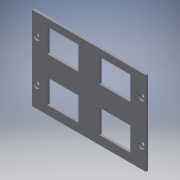
# Autodesk Inventor part: Ra-Manager_Painel-Placas_Tras_Plugs
Saved by Autodesk Inventor 2019.4 (Build 234330000, 330)
## iProperties
Created: 2020-03-24
Part Number: Ra-Manager_Painel-Placas_Tras_Plugs
Material: Genérico
Document SubType Name: Modeling
Designer: caiom
Density: 1 g/cm^3
Appearance: Padrão
Author: caiom
Autodesk Inventor part; units mm, degrees
ref_plane "YZ Plane" through (0, 0, 0) normal (1, 0, 0) x (0, 1, 0)
ref_plane "XZ Plane" through (0, 0, 0) normal (0, 1, 0) x (-1, 0, 0)
ref_plane "XY Plane" through (0, 0, 0) normal (0, 0, 1) x (1, 0, 0)
sketch "Esboço1" plane through (0, 0, 0) normal (0, 0, 1) x (1, 0, 0)
  line L0 (-50.5, -37) -> (50.5, -37)
  line L1 (50.5, -37) -> (50.5, 37)
  line L2 (50.5, 37) -> (-50.5, 37)
  line L3 (-50.5, 37) -> (-50.5, -37)
  point P0 (0, 0)
  point P1 (0, 0)
  dimension "d17" = 101
  dimension "d18" = 74
  dimension "d19" = 50.5
  dimension "d20" = 37
  dimension "d21" = 50.5
  dimension "d22" = 37
  constraints: 8 end point, 2 parallel, 1 perpendicular, 1 vertical
  measures "d17" distance between parallel lines of L1 L3
  measures "d18" distance between parallel lines of L0 L2
  measures "d19" distance from line of point (0, 0) L1
  measures "d20" distance from line of point (0, 0) L2
  measures "d21" distance from line of point (0, 0) L1
  measures "d22" distance from line of point (0, 0) L2
extrude "Extrusão1" add sketch "Esboço1" against normal blind 2
sketch "Esboço2" plane through (0, 0, 0) normal (0, 0, 1) x (1, 0, 0)
  line L0 (-50.5, -37) -> (-50.5, 37)
  line L1 (-50.5, 37) -> (50.5, 37)
  line L2 (-46.5, 37) -> (-46.5, -37) construction
  line L3 (50.5, -37) -> (-50.5, -37)
  line L4 (46.5, 37) -> (46.5, -37) construction
  line L5 (-50.5, 18.5) -> (50.5, 18.5) construction
  line L6 (-50.5, -18.5) -> (50.5, -18.5) construction
  line L7 (50.5, 37) -> (50.5, -37)
  point P0 (0, 0)
  point P1 (0, 0)
  point P2 (-46.5, 18.5)
  point P3 (-46.5, -18.5)
  point P4 (46.5, -18.5)
  point P5 (46.5, 18.5)
  dimension "d28" = 4
  dimension "d29" = 97
  dimension "d30" = 101
  dimension "d31" = 55.5
  dimension "d32" = 18.5
  dimension "d33" = 74
  dimension "d34" = 50.5
  dimension "d35" = 37
  dimension "d36" = 0
  constraints: 16 end point, 15 point on line, 5 parallel, 2 horizontal, 1 perpendicular
  measures "d28" distance between parallel lines of L7 L4
  measures "d29" distance between parallel lines of L7 L2
  measures "d30" distance between parallel lines of L7 L0
  measures "d31" distance between parallel lines of L5 L3
  measures "d32" distance between parallel lines of L6 L3
  measures "d33" distance between parallel lines of L1 L3
  measures "d34" distance from line of point (0, 0) L7
  measures "d35" distance from line of point (0, 0) L3
  measures "d36" distance from line of L5.end L7
hole "Furo1" at (-46.5, 18.5, 0) at (-46.5, -18.5, 0) at (46.5, -18.5, 0) at (46.5, 18.5, 0) direction (0, 0, -1) diameter 2.459 end through all counterbore diameter 6.5 counterbore depth 1.5
sketch "Esboço3" plane through (0, 0, -2) normal (0, 0, -1) x (-1, 0, 0)
  line L0 (-36.25, 14.25) -> (-36.25, 21.4827) projected
  line L1 (-36.0982, 21.8416) -> (-33.0537, 24.7952) projected
  line L2 (-32.75, 25.5129) -> (-32.75, 29.7) projected
  line L3 (-32.25, 30.2) -> (-13.75, 30.2) projected
  line L4 (-10.25, 14.25) -> (-10.25, 21.4827) projected
  line L5 (-12.9463, 24.7952) -> (-9.9018, 21.8416) projected
  line L6 (-13.25, 29.7) -> (-13.25, 25.5129) projected
  line L7 (-27.134, 10.7) -> (-18.866, 10.7) projected
  line L8 (-13.8, 11.25) -> (-32.2, 11.25) projected
  line L9 (-13.8, 10.2) -> (-32.2, 10.2) projected
  arc A0 (-36.25, 14.25) -> (-32.2, 10.2) centre (-32.2, 14.25) ccw projected
  line L10 (-36.25, 14.25) -> (-36.25, 21.4827) projected
  arc A1 (-13.8, 10.2) -> (-9.75, 14.25) centre (-13.8, 14.25) ccw projected
  line L11 (-9.75, 21.4827) -> (-9.75, 14.25) projected
  line L12 (-12.9463, 24.7952) -> (-9.9018, 21.8416) projected
  line L13 (-32.25, 30.2) -> (-13.75, 30.2) projected
  line L14 (-13.25, 29.7) -> (-13.25, 25.5129) projected
  arc A2 (-13.25, 29.7) -> (-13.75, 30.2) centre (-13.75, 29.7) ccw projected
  arc A3 (-13.25, 25.5129) -> (-12.9463, 24.7952) centre (-12.25, 25.5129) ccw projected
  arc A4 (-9.75, 21.4827) -> (-9.9018, 21.8416) centre (-10.25, 21.4827) ccw projected
  arc A5 (-32.25, 30.2) -> (-32.75, 29.7) centre (-32.25, 29.7) ccw projected
  arc A6 (-36.0982, 21.8416) -> (-36.25, 21.4827) centre (-35.75, 21.4827) ccw projected
  arc A7 (-33.0537, 24.7952) -> (-32.75, 25.5129) centre (-33.75, 25.5129) ccw projected
  line L15 (-36.75, 9.7) -> (-9.25, 9.7)
  line L16 (-9.25, 9.7) -> (-9.25, 30.7)
  line L17 (-9.25, 30.7) -> (-36.75, 30.7)
  line L18 (-36.75, 9.7) -> (-36.75, 30.7)
  line L19 (9.75, 14.25) -> (9.75, 21.4827) projected
  arc A8 (9.75, 14.25) -> (13.8, 10.2) centre (13.8, 14.25) ccw projected
  line L20 (32.2, 10.2) -> (13.8, 10.2) projected
  arc A9 (32.903, 10.7703) -> (35.75, 14.25) centre (32.2, 14.25) ccw projected
  arc A10 (32.2, 10.2) -> (36.25, 14.25) centre (32.2, 14.25) ccw projected
  line L21 (36.25, 21.4827) -> (36.25, 14.25) projected
  line L22 (13.75, 30.2) -> (32.25, 30.2) projected
  line L23 (-36.25, -24.75) -> (-36.25, -17.5173) projected
  arc A11 (-36.25, -24.75) -> (-32.2, -28.8) centre (-32.2, -24.75) ccw projected
  line L24 (-13.8, -28.8) -> (-32.2, -28.8) projected
  arc A12 (-13.8, -28.8) -> (-9.75, -24.75) centre (-13.8, -24.75) ccw projected
  line L25 (-9.75, -17.5173) -> (-9.75, -24.75) projected
  line L26 (-32.25, -8.8) -> (-13.75, -8.8) projected
  line L27 (13.75, -8.8) -> (32.25, -8.8) projected
  line L28 (9.75, -24.75) -> (9.75, -17.5173) projected
  arc A13 (9.75, -24.75) -> (13.8, -28.8) centre (13.8, -24.75) ccw projected
  line L29 (32.2, -28.8) -> (13.8, -28.8) projected
  arc A14 (32.2, -28.8) -> (36.25, -24.75) centre (32.2, -24.75) ccw projected
  line L30 (36.25, -17.5173) -> (36.25, -24.75) projected
  line L31 (9.25, 30.7) -> (36.75, 30.7)
  line L32 (36.75, 30.7) -> (36.75, 9.7)
  line L33 (36.75, 9.7) -> (9.25, 9.7)
  line L34 (9.25, 9.7) -> (9.25, 30.7)
  line L35 (-36.75, -8.3) -> (-36.75, -29.3)
  line L36 (-36.75, -29.3) -> (-9.25, -29.3)
  line L37 (-9.25, -29.3) -> (-9.25, -8.3)
  line L38 (-9.25, -8.3) -> (-36.75, -8.3)
  line L39 (9.25, -8.3) -> (9.25, -29.3)
  line L40 (9.25, -29.3) -> (36.75, -29.3)
  line L41 (36.75, -29.3) -> (36.75, -8.3)
  line L42 (36.75, -8.3) -> (9.25, -8.3)
  point P0 (0, 0)
  dimension "d51" = 1
  dimension "d52" = 27
  dimension "d53" = 19.45
  dimension "d54" = 1.55
  dimension "d67" = 0.5
  dimension "d68" = 0.5
  dimension "d69" = 27
  dimension "d70" = 27
  dimension "d71" = 45.5
  dimension "d72" = 73
  dimension "d73" = 20.5
  dimension "d74" = 0.5
  dimension "d75" = 18.5
  dimension "d76" = 39.5
  dimension "d77" = 18.5
  dimension "d78" = 0.5
  constraints: 32 end point, 8 perpendicular, 5 parallel, 2 horizontal, 1 vertical
  measures "d51" distance between parallel lines of L4 L16
  measures "d52" distance between parallel lines of L11 L18
  measures "d53" distance between parallel lines of L8 L17
  measures "d54" distance between parallel lines of L8 L15
  measures "d67" distance between parallel lines of L21 L32
  measures "d68" distance between parallel lines of L21 L41
  measures "d69" distance between parallel lines of L21 L34
  measures "d70" distance between parallel lines of L21 L39
  measures "d71" distance between parallel lines of L21 L37
  measures "d72" distance between parallel lines of L21 L35
  measures "d73" distance between parallel lines of L20 L31
  measures "d74" distance between parallel lines of L20 L33
  measures "d75" distance between parallel lines of L20 L42
  measures "d76" distance between parallel lines of L20 L40
  measures "d77" distance between parallel lines of L20 L38
  measures "d78" distance between parallel lines of L29 L36
extrude "Extrusão3" cut sketch "Esboço3" against normal blind 10 contours L0 A6 L1 A7 L2 A5 L3 A2 L6 A3 L5 A4 L11 A1 L9 A0 | L18 L17 L16 L15 | L31 L32 L33 L34 | L38 L37 L36 L35 | L42 L41 L40 L39
